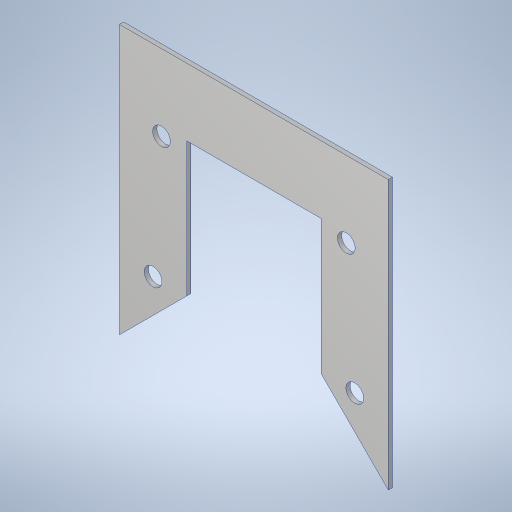
# Autodesk Inventor part: AI1-001
Saved by Autodesk Inventor 2023.4 (Build 274418000, 418)
## iProperties
Created: 2025-01-15
Part Number: AI1-001
Material: Aluminum 6061
Document SubType Name: Modeling
Designer: mavericks
Density: 2.7 g/cm^3
Appearance: Aluminum - Flat
Author: mavericks
Autodesk Inventor part; units mm, degrees
ref_plane "YZ Plane" through (0, 0, 0) normal (1, 0, 0) x (0, 1, 0)
ref_plane "XZ Plane" through (0, 0, 0) normal (0, 1, 0) x (-1, 0, 0)
ref_plane "XY Plane" through (0, 0, 0) normal (0, 0, 1) x (1, 0, 0)
sketch "Sketch1" plane through (0, 0, 0) normal (0, 0, 1) x (1, 0, 0)
  line L0 (-203.2, 203.2) -> (203.2, 203.2)
  line L1 (203.2, 203.2) -> (203.2, -203.2)
  line L2 (-203.2, -203.2) -> (-203.2, 203.2)
  line L3 (-203.2, 203.2) -> (203.2, -203.2) construction
  line L4 (203.2, 203.2) -> (-203.2, -203.2) construction
  line L5 (-203.2, -203.2) -> (-101.6, -101.6)
  line L6 (-101.6, -101.6) -> (-101.6, 101.6)
  line L7 (-101.6, 101.6) -> (101.6, 101.6)
  line L8 (101.6, 101.6) -> (101.6, -101.6)
  line L9 (203.2, -203.2) -> (101.6, -101.6)
  point P0 (0, 0)
  dimension "d1" = 406.4
  dimension "d2" = 101.6
  dimension "d3" = 101.6
  constraints: 20 end point, 4 point on line, 3 perpendicular, 2 midpoint, 1 collinear, 1 horizontal, 1 parallel, 1 vertical
  measures "d1" distance of L0.end L1.end
  measures "d2" distance between parallel lines of L6 L2
  measures "d3" distance between parallel lines of L0 L7
extrude "Extrusion1" add sketch "Sketch1" along normal blind 6.35
sketch "Sketch2" plane through (0, 0, 6.35) normal (0, 0, 1) x (1, 0, 0)
  line L0 (-101.6, -101.6) -> (-101.6, 101.6) projected
  line L1 (101.6, 101.6) -> (101.6, -101.6) projected
  point P0 (0, 0)
  point P1 (-152.4, -101.6)
  point P2 (-139.7, 88.4462)
  point P3 (139.7, 88.4462)
  point P4 (152.4, -101.6)
  dimension "d6" = 50.8
  dimension "d7" = 38.1
  dimension "d8" = 38.1
  dimension "d9" = 50.8
  constraints: 2 horizontal alignment
  measures "d6" distance from line of L0 point (-152.4, -101.6)
  measures "d7" distance from line of L0 point (-139.7, 88.446)
  measures "d8" distance from line of L1 point (139.7, 88.446)
  measures "d9" distance from line of L1 point (152.4, -101.6)
hole "Hole1" at (-152.4, -101.6, 6.35) at (-139.7, 88.4462, 6.35) at (139.7, 88.4462, 6.35) at (152.4, -101.6, 6.35) direction (0, 0, -1) diameter 26.9875 end through all
equation "\"d8\" = d7"
equation "\"d9\" = d6"
body "Solid1"
